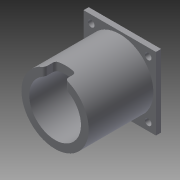
# Autodesk Inventor part: 000114
Saved by Autodesk Inventor 2015 (Build 190159000, 159)
## iProperties
Created: 2015-05-13
Part Number: 000114
Material: Generic
Document SubType Name: Modeling
Designer: Wesley
Density: 1 g/cm^3
Appearance: Default
Author: Wesley
Autodesk Inventor part; units mm, degrees
ref_plane "YZ Plane" through (0, 0, 0) normal (1, 0, 0) x (0, 1, 0)
ref_plane "XY Plane" through (0, 0, 0) normal (0, 0, 1) x (1, 0, 0)
sketch "Sketch1" plane through (0, 0, 0) normal (0, 0, 1) x (1, 0, 0)
  line L0 (17.78, 17.78) -> (-17.78, 17.78)
  line L1 (-17.78, 17.78) -> (-17.78, -17.78)
  line L2 (-17.78, -17.78) -> (17.78, -17.78)
  line L3 (17.78, -17.78) -> (17.78, 17.78)
  point P0 (0, 0)
  dimension "d0" = 35.56
  dimension "d1" = 35.56
  dimension "d2" = 17.78
  dimension "d3" = 17.78
  constraints: 8 end point, 2 parallel, 1 horizontal, 1 perpendicular
  measures "d0" distance of L2.end L1.end
  measures "d1" distance of L1.end L0.end
  measures "d2" distance from line of L0 point (0, 0)
  measures "d3" distance from line of L3 point (0, 0)
extrude "Extrusion1" add sketch "Sketch1" along normal blind 2.54
sketch "Sketch2" plane through (0, 0, 2.54) normal (0, 0, 1) x (1, 0, 0)
  circle A0 centre (0, 0) radius 12.7
  circle A1 centre (0, 0) radius 16.51
  dimension "d6" = 25.4
  dimension "d7" = 3.81
  constraints: 2 centre point, 1 coincident
  measures "d6" diameter of A0
  measures "d7" radial gap between concentric circles of A0 A1
extrude "Extrusion2" add sketch "Sketch2" along normal blind 31.75
sketch "Sketch3" plane through (0, 0, 2.54) normal (0, 0, 1) x (1, 0, 0)
  line L0 (17.78, 17.78) -> (-17.78, 17.78) projected
  line L1 (-17.78, 17.78) -> (-17.78, -17.78) projected
  line L2 (17.78, -17.78) -> (17.78, 17.78) projected
  line L3 (-17.78, -17.78) -> (17.78, -17.78) projected
  point P0 (0, 0)
  point P1 (-13.97, -13.97)
  point P2 (13.97, -13.97)
  point P3 (13.97, 13.97)
  point P4 (-13.97, 13.97)
  dimension "d10" = 3.81
  dimension "d11" = 3.81
  dimension "d12" = 3.81
  dimension "d13" = 3.81
  dimension "d14" = 3.81
  dimension "d15" = 3.81
  dimension "d16" = 3.81
  dimension "d17" = 3.81
  measures "d10" distance from line of L0 point (-13.97, 13.97)
  measures "d11" distance from line of L1 point (-13.97, 13.97)
  measures "d12" distance from line of L0 point (13.97, 13.97)
  measures "d13" distance from line of L2 point (13.97, 13.97)
  measures "d14" distance from line of L3 point (13.97, -13.97)
  measures "d15" distance from line of L2 point (13.97, -13.97)
  measures "d16" distance from line of L1 point (-13.97, -13.97)
  measures "d17" distance from line of L3 point (-13.97, -13.97)
hole "Hole1" at (-13.97, -13.97, 2.54) at (13.97, -13.97, 2.54) at (13.97, 13.97, 2.54) at (-13.97, 13.97, 2.54) direction (0, 0, -1) diameter 3.175 depth 3.175 tip angle 118
ref_plane "Work Plane1" through (0, 16.51, 0) normal (0, 1, 0) x (-1, 0, 0)
sketch "Sketch4" plane through (0, 16.51, 0) normal (0, 1, 0) x (-1, 0, 0)
  line L0 (-12.7, 34.29) -> (12.7, 34.29) projected
  line L1 (5.08, 34.29) -> (-5.08, 34.29)
  line L2 (-5.08, 34.29) -> (-5.08, 29.21)
  line L3 (-5.08, 29.21) -> (5.08, 29.21)
  line L4 (5.08, 29.21) -> (5.08, 34.29)
  line L5 (0, -6.858) -> (0, 41.148) projected
  point P0 (0, 0)
  dimension "d26" = 5.08
  dimension "d27" = 10.16
  dimension "d28" = 5.08
  constraints: 8 end point, 2 parallel, 1 horizontal, 1 perpendicular, 1 point on line
  measures "d26" distance of L1.end L2.end
  measures "d27" distance of L2.end L3.end
  measures "d28" distance between parallel lines of L2 L5
extrude "Extrusion3" cut sketch "Sketch4" against normal blind 10.16
sketch "Sketch5" plane through (0, 0, 2.54) normal (0, 0, 1) x (1, 0, 0)
  circle A0 centre (0, 0) radius 4.445
  dimension "d31" = 8.89
  constraints: 1 centre point, 1 coincident
  measures "d31" diameter of A0
extrude "Extrusion4" cut sketch "Sketch5" against normal through all
fillet "Fillet1" radius 1.27 4 edges at (-5.08, 13.6744, 29.21) (-5.08, 13.6744, 34.29) (5.08, 13.6744, 34.29) (5.08, 13.6744, 29.21)
body "Solid1"
